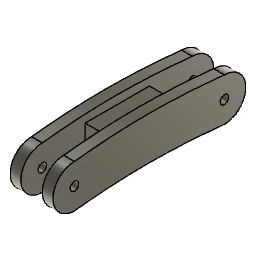
arm1 v1 (Autodesk Fusion 360 design; units mm, degrees)
Autodesk Fusion 360 part; units mm, degrees
sketch "Sketch1" plane through (0, 0, 0) normal (1, 0, 0) x (0, 1, 0)
  spline S0 degree 5 poles (0, 50) (6.8077, 50.7622) (20.44, 52.2195) (40.9391, 54.2045) (68.3744, 56.4426) (102.852, 58.5132) (137.5289, 59.7935) (172.421, 60.2212) (207.5356, 59.7669) (242.8628, 58.4704) (278.3858, 56.3974) (306.9479, 54.1699) (328.445, 52.1996) (342.8095, 50.755) (350, 50) knots 0 0 0 0 0 0 0.1 0.2 0.3 0.4 0.5 0.6 0.7 0.8 0.9 1 1 1 1 1 1
  spline S1 degree 5 poles (0, -50) (6.8077, -49.2378) (20.44, -47.7805) (40.9391, -45.7955) (68.3744, -43.5574) (102.852, -41.4868) (137.5289, -40.2065) (172.421, -39.7788) (207.5356, -40.2331) (242.8628, -41.5296) (278.3858, -43.6026) (306.9479, -45.8301) (328.445, -47.8004) (342.8095, -49.245) (350, -50) knots 0 0 0 0 0 0 0.1 0.2 0.3 0.4 0.5 0.6 0.7 0.8 0.9 1 1 1 1 1 1
  arc A0 (0, 50) -> (10.7493, -48.8308) centre (0, 0) ccw
  circle A1 centre (0, 0) radius 10
  circle A2 centre (350, 0) radius 10
  arc A3 (339.8569, -48.9604) -> (350, 50) centre (350, 0) ccw
  point P0 (170, 60)
  point P1 (170, -40)
  dimension "d1" = 100
  dimension "d2" = 350
  dimension "d3" = 100
  dimension "d4" = 20
  dimension "d5" = 20
  constraint coincident A0.centre A1.centre
  constraint coincident S1.end A3
  constraint coincident S1 A0.end
  constraint concentric A0 A1
  constraint concentric A2 A3
  constraint coincident S1 A3.start
  measures "d1" diameter of A0
  measures "d2" distance of S0.start S0.end
  measures "d3" distance of S0.start S1.start
  measures "d4" diameter of A1
  measures "d5" diameter of A2
extrude "Extrude1" add sketch "Sketch1" along normal blind 25 contours S0 S1 A0 A3
sketch "Sketch2" plane through (25, 0, 0) normal (1, 0, 0) x (0, 1, 0)
  circle A0 centre (350, 0) radius 10
  circle A1 centre (0, 0) radius 10
  arc A2 (0, 50) -> (0, -50) centre (0, 0) ccw
  spline S0 degree 5 poles (0, -50) (2.1482, -49.7595) (4.2972, -49.5223) (6.4471, -49.2885) (8.5978, -49.058) (10.7493, -48.8308) knots 0 0 0 0 0 0 0.031555 0.031555 0.031555 0.031555 0.031555 0.031555
  spline S1 degree 5 poles (10.7493, -48.8308) (15.4162, -48.3381) (26.9111, -47.1643) (45.2687, -45.446) (70.5503, -43.4268) (102.852, -41.4868) (137.5289, -40.2065) (172.421, -39.7788) (207.5356, -40.2331) (242.8628, -41.5296) (276.3801, -43.4855) (302.9169, -45.5185) (322.3782, -47.2522) (334.703, -48.445) (339.8569, -48.9604) knots 0.031555 0.031555 0.031555 0.031555 0.031555 0.031555 0.1 0.2 0.3 0.4 0.5 0.6 0.7 0.8 0.9 0.971769 0.971769 0.971769 0.971769 0.971769 0.971769
  spline S2 degree 5 poles (339.8569, -48.9604) (341.8842, -49.1631) (343.9121, -49.3684) (345.9408, -49.5763) (347.9701, -49.7868) (350, -50) knots 0.971769 0.971769 0.971769 0.971769 0.971769 0.971769 1 1 1 1 1 1
  arc A3 (350, -50) -> (350, 50) centre (350, 0) ccw
  spline S3 degree 5 poles (350, 50) (342.8095, 50.755) (328.445, 52.1996) (306.9479, 54.1699) (278.3858, 56.3974) (242.8628, 58.4704) (207.5356, 59.7669) (172.421, 60.2212) (137.5289, 59.7935) (102.852, 58.5132) (68.3744, 56.4426) (40.9391, 54.2045) (20.44, 52.2195) (6.8077, 50.7622) (0, 50) knots -1 -1 -1 -1 -1 -1 -0.9 -0.8 -0.7 -0.6 -0.5 -0.4 -0.3 -0.2 -0.1 0 0 0 0 0 0
  line L0 (100, 40) -> (250, 40)
  line L1 (250, 40) -> (250, -20)
  line L2 (250, -20) -> (100, -20)
  line L3 (100, -20) -> (100, 40)
  constraint horizontal L0
  constraint vertical L1
  constraint horizontal L2
  constraint vertical L3
extrude "Extrude2" add sketch "Sketch2" along normal blind 25 contours L0 L1 L2 L3
move_body "Move1" bodies 1 to x (1, 0, 0) y (0, 1, 0) z (0, 0, 1) at (-50, 0, 0)
mirror "Mirror1" about plane through (0, 0, 0) normal (1, 0, 0) of bodies 1 merged
